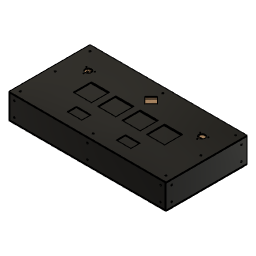
OpenSDVX Con v2 (Autodesk Fusion 360 design; units mm, degrees)
Autodesk Fusion 360 part; units mm, degrees
(part 1 of 2)
sketch "Bottom Panel Profile Sketch" plane through (0, 0, 0) normal (0, 1, 0) x (1, 0, 0) in component "Box"
  line L0 (245, 125) -> (-245, 125)
  line L1 (-245, 125) -> (-245, -125)
  line L2 (-245, -125) -> (245, -125)
  line L3 (245, -125) -> (245, 125)
  line L4 (245, 125) -> (-245, -125) construction
  line L5 (-245, 125) -> (245, -125) construction
  dimension "d31" = 490
  dimension "d32" = 250
  constraint horizontal L0
  constraint perpendicular L0 L1
  constraint parallel L0 L2
  constraint parallel L1 L3
  constraint coincident L4 origin
  constraint coincident L5 origin
  measures "d31" distance of L1.end L2.end
  measures "d32" distance of L0.end L1.end
extrude "Extrude1" add sketch "Bottom Panel Profile Sketch" along normal blind 6 makes body 1 in component "Box"
sketch "Bottom Panel Front Fingers Sketch" plane through (0, 0, 125) normal (0, 0, 1) x (1, 0, 0) in component "Box"
  line L0 (-245, 0) -> (245, 0)
  line L1 (245, 0) -> (245, 6)
  line L2 (245, 6) -> (-245, 6)
  line L3 (-245, 6) -> (-245, 0)
  line L4 (0, 6) -> (0, 0) construction
  line L5 (-232.4359, 3) -> (232.4359, 3) construction
  line L6 (-232.4359, 0) -> (-219.8718, 0)
  line L7 (-219.8718, 0) -> (-219.8718, 6)
  line L8 (-219.8718, 6) -> (-232.4359, 6)
  line L9 (-232.4359, 6) -> (-232.4359, 0)
  dimension "d35" = 12.5641
  dimension "d36" = 464.8718
  constraint midpoint L2 L4.start
  constraint coincident L4.end origin
  constraint perpendicular L4 L5
  constraint midpoint L4 L5
  constraint horizontal L6
  constraint vertical L7
  constraint horizontal L8
  constraint vertical L9
  constraint coincident L2 L7.end
  constraint coincident L0 L6.start
  constraint coincident L5.start L9
  measures "d35" distance of L7.end L8.end
  measures "d36" distance of L5.start L5.end
extrude "Extrude2" cut sketch "Bottom Panel Front Fingers Sketch" against normal blind 6 contours L0 L2 L6 L7 L8 L9 bodies 1 in component "Box"
pattern_linear "R-Pattern1" count 19 spacing 25.1282 along (1, 0, 0) count 2 spacing 244 along (0, 0, -1) of "Extrude2" in component "Box"
sketch "Bottom Panel Left Fingers Sketch" plane through (-245, 0, 0) normal (-1, 0, 0) x (0, 0, 1) in component "Box"
  line L0 (-125, 0) -> (125, 0)
  line L1 (125, 0) -> (125, 6)
  line L2 (125, 6) -> (-125, 6)
  line L3 (-125, 6) -> (-125, 0)
  line L4 (0, 6) -> (0, 0) construction
  line L5 (-111.8421, 3) -> (111.8421, 3) construction
  line L6 (98.6842, 0) -> (111.8421, 0)
  line L7 (111.8421, 0) -> (111.8421, 6)
  line L8 (111.8421, 6) -> (98.6842, 6)
  line L9 (98.6842, 6) -> (98.6842, 0)
  dimension "d43" = 13.1579
  dimension "d44" = 223.6842
  constraint midpoint L2 L4.start
  constraint coincident L4.end origin
  constraint perpendicular L4 L5
  constraint midpoint L4 L5
  constraint horizontal L6
  constraint vertical L7
  constraint horizontal L8
  constraint vertical L9
  constraint coincident L2 L7.end
  constraint coincident L0 L6.start
  constraint coincident L5.end L7
  measures "d43" distance of L6.start L6.end
  measures "d44" distance of L5.start L5.end
extrude "Extrude3" cut sketch "Bottom Panel Left Fingers Sketch" against normal blind 6 contours L0 L2 L6 L7 L8 L9 bodies 1 in component "Box"
pattern_linear "R-Pattern2" count 9 spacing 26.3158 along (0, 0, -1) count 2 spacing 484 along (1, 0, 0) of "Extrude3" in component "Box"
sketch "Front Panel Front Fingers Sketch" plane through (0, 0, 125) normal (0, 0, 1) x (1, 0, 0) in component "Box"
  line L0 (-232.4359, 0) -> (-232.4359, 6)
  line L1 (-232.4359, 6) -> (-245, 6)
  line L2 (-245, 6) -> (-245, 0)
  line L3 (-245, 0) -> (-232.4359, 0)
  line L4 (-245, 0) -> (245, 0)
  line L5 (245, 0) -> (245, 74)
  line L6 (245, 74) -> (-245, 74)
  line L7 (-245, 74) -> (-245, 0)
  dimension "d51" = 490
  dimension "d52" = 74
  constraint horizontal L4
  constraint vertical L5
  constraint horizontal L6
  constraint vertical L7
  constraint coincident L2.end L3.start
  measures "d51" distance of L2.end L4.end
  measures "d52" distance of L2.end L6.end
extrude "Extrude4" add sketch "Front Panel Front Fingers Sketch" against normal blind 6 separate body contours L0 L1 L4 L5 L6 L7 makes body 2 in component "Box"
combine "Combine1" operation cut target body 2 tool bodies 1 keep tools in component "Box"
sketch "Front Panel Left Finger Sketch" plane through (0, 0, 125) normal (0, 0, 1) x (1, 0, 0) in component "Box"
  line L0 (232.4359, 6) -> (245, 6)
  line L1 (245, 6) -> (245, 74)
  line L2 (245, 74) -> (-245, 74)
  line L3 (-245, 74) -> (-245, 6)
  line L4 (-245, 6) -> (-232.4359, 6)
  line L5 (-232.4359, 6) -> (-232.4359, 0)
  line L6 (-232.4359, 0) -> (-219.8718, 0)
  line L7 (-219.8718, 0) -> (-219.8718, 6)
  line L8 (-219.8718, 6) -> (-207.3077, 6)
  line L9 (-207.3077, 6) -> (-207.3077, 0)
  line L10 (-207.3077, 0) -> (-194.7436, 0)
  line L11 (-194.7436, 0) -> (-194.7436, 6)
  line L12 (-194.7436, 6) -> (-182.1795, 6)
  line L13 (-182.1795, 6) -> (-182.1795, 0)
  line L14 (-182.1795, 0) -> (-169.6154, 0)
  line L15 (-169.6154, 0) -> (-169.6154, 6)
  line L16 (-169.6154, 6) -> (-157.0513, 6)
  line L17 (-157.0513, 6) -> (-157.0513, 0)
  line L18 (-157.0513, 0) -> (-144.4872, 0)
  line L19 (-144.4872, 0) -> (-144.4872, 6)
  line L20 (-144.4872, 6) -> (-131.9231, 6)
  line L21 (-131.9231, 6) -> (-131.9231, 0)
  line L22 (-131.9231, 0) -> (-119.359, 0)
  line L23 (-119.359, 0) -> (-119.359, 6)
  line L24 (-119.359, 6) -> (-106.7949, 6)
  line L25 (-106.7949, 6) -> (-106.7949, 0)
  line L26 (-106.7949, 0) -> (-94.2308, 0)
  line L27 (-94.2308, 0) -> (-94.2308, 6)
  line L28 (-94.2308, 6) -> (-81.6667, 6)
  line L29 (-81.6667, 6) -> (-81.6667, 0)
  line L30 (-81.6667, 0) -> (-69.1026, 0)
  line L31 (-69.1026, 0) -> (-69.1026, 6)
  line L32 (-69.1026, 6) -> (-56.5385, 6)
  line L33 (-56.5385, 6) -> (-56.5385, 0)
  line L34 (-56.5385, 0) -> (-43.9744, 0)
  line L35 (-43.9744, 0) -> (-43.9744, 6)
  line L36 (-43.9744, 6) -> (-31.4103, 6)
  line L37 (-31.4103, 6) -> (-31.4103, 0)
  line L38 (-31.4103, 0) -> (-18.8462, 0)
  line L39 (-18.8462, 0) -> (-18.8462, 6)
  line L40 (-18.8462, 6) -> (-6.2821, 6)
  line L41 (-6.2821, 6) -> (-6.2821, 0)
  line L42 (-6.2821, 0) -> (6.2821, 0)
  line L43 (6.2821, 0) -> (6.2821, 6)
  line L44 (6.2821, 6) -> (18.8462, 6)
  line L45 (18.8462, 6) -> (18.8462, 0)
  line L46 (18.8462, 0) -> (31.4103, 0)
  line L47 (31.4103, 0) -> (31.4103, 6)
  line L48 (-245, 40) -> (-239, 40) construction
  line L49 (-242, 62.2) -> (-242, 17.8) construction
  line L50 (-245, 32.6) -> (-239, 32.6)
  line L51 (-239, 32.6) -> (-239, 17.8)
  line L52 (-239, 17.8) -> (-245, 17.8)
  line L53 (-245, 17.8) -> (-245, 32.6)
  line L54 (31.4103, 6) -> (43.9744, 6)
  line L55 (43.9744, 6) -> (43.9744, 0)
  line L56 (43.9744, 0) -> (56.5385, 0)
  line L57 (56.5385, 0) -> (56.5385, 6)
  line L58 (56.5385, 6) -> (69.1026, 6)
  line L59 (69.1026, 6) -> (69.1026, 0)
  line L60 (69.1026, 0) -> (81.6667, 0)
  line L61 (81.6667, 0) -> (81.6667, 6)
  line L62 (81.6667, 6) -> (94.2308, 6)
  line L63 (94.2308, 6) -> (94.2308, 0)
  line L64 (94.2308, 0) -> (106.7949, 0)
  line L65 (106.7949, 0) -> (106.7949, 6)
  line L66 (106.7949, 6) -> (119.359, 6)
  line L67 (119.359, 6) -> (119.359, 0)
  line L68 (119.359, 0) -> (131.9231, 0)
  line L69 (131.9231, 0) -> (131.9231, 6)
  line L70 (131.9231, 6) -> (144.4872, 6)
  line L71 (144.4872, 6) -> (144.4872, 0)
  line L72 (144.4872, 0) -> (157.0513, 0)
  line L73 (157.0513, 0) -> (157.0513, 6)
  line L74 (157.0513, 6) -> (169.6154, 6)
  line L75 (169.6154, 6) -> (169.6154, 0)
  line L76 (169.6154, 0) -> (182.1795, 0)
  line L77 (182.1795, 0) -> (182.1795, 6)
  line L78 (182.1795, 6) -> (194.7436, 6)
  line L79 (194.7436, 6) -> (194.7436, 0)
  line L80 (194.7436, 0) -> (207.3077, 0)
  line L81 (207.3077, 0) -> (207.3077, 6)
  line L82 (207.3077, 6) -> (219.8718, 6)
  line L83 (219.8718, 6) -> (219.8718, 0)
  line L84 (219.8718, 0) -> (232.4359, 0)
  line L85 (232.4359, 0) -> (232.4359, 6)
  dimension "d55" = 6
  dimension "d56" = 14.8
  dimension "d57" = 44.4
  constraint midpoint L3 L48.start
  constraint perpendicular L3 L48
  constraint perpendicular L48 L49
  constraint midpoint L48 L49
  constraint horizontal L50
  constraint vertical L51
  constraint horizontal L52
  constraint vertical L53
  constraint coincident L3 L50.start
  constraint coincident L49.end L52
  constraint coincident L48.end L51
  measures "d55" distance of L48.start L48.end
  measures "d56" distance of L50.start L52.end
  measures "d57" distance of L49.start L49.end
extrude "Extrude5" cut sketch "Front Panel Left Finger Sketch" against normal blind 6 contours L3 L50 L51 L52 L53 bodies 2 in component "Box"
pattern_linear "R-Pattern3" count 2 spacing 29.6 along (0, 1, 0) count 2 spacing 484 along (1, 0, 0) of "Extrude5" in component "Box"
pattern_linear "R-Pattern6" count 2 spacing 68 along (0, 1, 0) of bodies 1 makes body 3 in component "Box"
combine "Combine3" operation cut target body 2 tool bodies 3 keep tools in component "Box"
pattern_linear "R-Pattern7" count 2 spacing 244 along (0, 0, -1) of bodies 2 makes body 4 in component "Box"
sketch "Left Panel Profile Sketch" plane through (-245, 0, 0) normal (-1, 0, 0) x (0, 0, 1) in component "Box"
  line L0 (111.8421, 6) -> (111.8421, 0)
  line L1 (111.8421, 0) -> (125, 0)
  line L2 (125, 0) -> (125, 6)
  line L3 (125, 6) -> (111.8421, 6)
  line L4 (125, 0) -> (-125, 0)
  line L5 (-125, 0) -> (-125, 74)
  line L6 (-125, 74) -> (125, 74)
  line L7 (125, 74) -> (125, 0)
  dimension "d88" = 250
  dimension "d89" = 74
  constraint horizontal L4
  constraint vertical L5
  constraint horizontal L6
  constraint vertical L7
  constraint coincident L1.end L2.start
  measures "d88" distance of L1.end L4.end
  measures "d89" distance of L1.end L6.end
extrude "Extrude8" add sketch "Left Panel Profile Sketch" against normal blind 6 separate body contours L0 L3 L4 L5 L6 L7 makes body 5 in component "Box"
combine "Combine4" operation cut target body 5 tool bodies 3 2 4 1 keep tools in component "Box"
pattern_linear "R-Pattern8" count 2 spacing 484 along (1, 0, 0) of bodies 5 makes body 6 in component "Box"
sketch "Bottom Plate Profile Sketch" plane through (0, 0, 0) normal (0, 1, 0) x (1, 0, 0) in component "Box"
  line L0 (248, 128) -> (-248, 128)
  line L1 (-248, 128) -> (-248, -128)
  line L2 (-248, -128) -> (248, -128)
  line L3 (248, -128) -> (248, 128)
  line L4 (248, 128) -> (-248, -128) construction
  line L5 (-248, 128) -> (248, -128) construction
  dimension "d100" = 496
  dimension "d101" = 256
  constraint horizontal L0
  constraint perpendicular L0 L1
  constraint parallel L0 L2
  constraint parallel L1 L3
  constraint coincident L4 origin
  constraint coincident L5 origin
  measures "d100" distance of L1.end L2.end
  measures "d101" distance of L0.end L1.end
extrude "Extrude10" add sketch "Bottom Plate Profile Sketch" against normal blind 3 separate body makes body 7 in component "Box"
pattern_linear "R-Pattern9" count 2 spacing 77 along (0, 1, 0) of bodies 7 makes body 8 in component "Box"
sketch "Left Plate Profile Sketch" plane through (-245, 0, 0) normal (-1, 0, 0) x (0, -1, 0) in component "Box"
  line L0 (0, 0) -> (-74, 0) construction
  line L1 (-37, -125) -> (-37, 125) construction
  line L2 (-74, 128) -> (0, 128)
  line L3 (0, 128) -> (0, -128)
  line L4 (0, -128) -> (-74, -128)
  line L5 (-74, -128) -> (-74, 128)
  line L6 (-74, 128) -> (0, -128) construction
  line L7 (0, 128) -> (-74, -128) construction
  point P0 (-37, 0)
  dimension "d115" = 74
  dimension "d116" = 250
  dimension "d117" = 74
  dimension "d118" = 256
  constraint coincident L0.start origin
  constraint horizontal L0
  constraint vertical L1
  constraint midpoint L0 L1
  constraint horizontal L2
  constraint perpendicular L2 L3
  constraint parallel L2 L4
  constraint parallel L3 L5
  constraint coincident L6 P0
  constraint coincident L7 P0
  constraint midpoint L0 P0
  measures "d115" distance of L0.start L0.end
  measures "d116" distance of L1.start L1.end
  measures "d117" distance of L3.end L4.end
  measures "d118" distance of L2.end L3.end
extrude "Extrude12" add sketch "Left Plate Profile Sketch" along normal blind 3 separate body makes body 9 in component "Box"
pattern_linear "R-Pattern10" count 2 spacing 493 along (1, 0, 0) of bodies 9 makes body 10 in component "Box"
sketch "Front Plate Profile Sketch" plane through (0, 0, 0) normal (0, 0, 1) x (1, 0, 0) in component "Box"
  line L0 (0, 0) -> (0, 74) construction
  line L1 (-245, 37) -> (245, 37)
  line L2 (245, 74) -> (-245, 74)
  line L3 (-245, 74) -> (-245, 0)
  line L4 (-245, 0) -> (245, 0)
  line L5 (245, 0) -> (245, 74)
  line L6 (245, 74) -> (-245, 0) construction
  line L7 (-245, 74) -> (245, 0) construction
  point P0 (0, 37)
  dimension "d125" = 74
  dimension "d126" = 490
  dimension "d127" = 490
  dimension "d128" = 74
  constraint coincident L0.start origin
  constraint vertical L0
  constraint perpendicular L0 L1
  constraint midpoint L0 L1
  constraint horizontal L2
  constraint perpendicular L2 L3
  constraint parallel L2 L4
  constraint parallel L3 L5
  constraint coincident L6 P0
  constraint coincident L7 P0
  constraint midpoint L1 P0
  measures "d125" distance of L0.start L0.end
  measures "d126" distance of L1.start L1.end
  measures "d127" distance of L3.end L4.end
  measures "d128" distance of L2.end L3.end
extrude "Extrude13" add sketch "Front Plate Profile Sketch" along normal blind 3 from surface at 125 separate body makes body 11 in component "Box"
pattern_linear "R-Pattern11" count 2 spacing 253 along (0, 0, -1) of bodies 11 makes body 12 in component "Box"
sketch "Top Plate Screws Sketch" plane through (0, 77, 0) normal (0, 1, 0) x (-1, 0, 0) in component "Box"
  line L0 (-248, 128) -> (-248, -128)
  line L1 (-248, -128) -> (248, -128)
  line L2 (248, -128) -> (248, 128)
  line L3 (248, 128) -> (-248, 128)
  circle A0 centre (230, -110) radius 2.5
  circle A1 centre (0, -110) radius 2.5
  circle A2 centre (230, 0) radius 2.5
  line L4 (226, -112.3094) -> (230, -114.6188)
  line L5 (230, -114.6188) -> (234, -112.3094)
  line L6 (234, -112.3094) -> (234, -107.6906)
  line L7 (234, -107.6906) -> (230, -105.3812)
  line L8 (230, -105.3812) -> (226, -107.6906)
  line L9 (226, -107.6906) -> (226, -112.3094)
  line L10 (4, -107.6906) -> (0, -105.3812)
  line L11 (0, -105.3812) -> (-4, -107.6906)
  line L12 (-4, -107.6906) -> (-4, -112.3094)
  line L13 (-4, -112.3094) -> (0, -114.6188)
  line L14 (4, -112.3094) -> (4, -107.6906)
  line L15 (0, -114.6188) -> (4, -112.3094)
  line L16 (-226, -107.6906) -> (-230, -105.3812)
  line L17 (-230, -105.3812) -> (-234, -107.6906)
  line L18 (-234, -107.6906) -> (-234, -112.3094)
  line L19 (-234, -112.3094) -> (-230, -114.6188)
  line L20 (-226, -112.3094) -> (-226, -107.6906)
  line L21 (-230, -114.6188) -> (-226, -112.3094)
  line L22 (234, 2.3094) -> (230, 4.6188)
  line L23 (230, 4.6188) -> (226, 2.3094)
  line L24 (226, 2.3094) -> (226, -2.3094)
  line L25 (226, -2.3094) -> (230, -4.6188)
  line L26 (234, -2.3094) -> (234, 2.3094)
  line L27 (230, -4.6188) -> (234, -2.3094)
  line L28 (-226, 2.3094) -> (-230, 4.6188)
  line L29 (-230, 4.6188) -> (-234, 2.3094)
  line L30 (-234, 2.3094) -> (-234, -2.3094)
  line L31 (-234, -2.3094) -> (-230, -4.6188)
  line L32 (-226, -2.3094) -> (-226, 2.3094)
  line L33 (-230, -4.6188) -> (-226, -2.3094)
  line L34 (234, 112.3094) -> (230, 114.6188)
  line L35 (230, 114.6188) -> (226, 112.3094)
  line L36 (226, 112.3094) -> (226, 107.6906)
  line L37 (226, 107.6906) -> (230, 105.3812)
  line L38 (234, 107.6906) -> (234, 112.3094)
  line L39 (230, 105.3812) -> (234, 107.6906)
  line L40 (4, 112.3094) -> (0, 114.6188)
  line L41 (0, 114.6188) -> (-4, 112.3094)
  line L42 (-4, 112.3094) -> (-4, 107.6906)
  line L43 (-4, 107.6906) -> (0, 105.3812)
  line L44 (4, 107.6906) -> (4, 112.3094)
  line L45 (0, 105.3812) -> (4, 107.6906)
  line L46 (-226, 112.3094) -> (-230, 114.6188)
  line L47 (-230, 114.6188) -> (-234, 112.3094)
  line L48 (-234, 112.3094) -> (-234, 107.6906)
  line L49 (-234, 107.6906) -> (-230, 105.3812)
  line L50 (-226, 107.6906) -> (-226, 112.3094)
  line L51 (-230, 105.3812) -> (-226, 107.6906)
  circle A3 centre (-230, -110) radius 2.5
  circle A4 centre (-230, 0) radius 2.5
  circle A5 centre (230, 110) radius 2.5
  circle A6 centre (0, 110) radius 2.5
  circle A7 centre (-230, 110) radius 2.5
  point P0 (230, -110)
  dimension "d136" = 5
  dimension "d137" = 18
  dimension "d138" = 18
  dimension "d141" = -460
  dimension "d142" = 220
  dimension "d201" = 4
  dimension "d202" = 90
  dimension "d205" = -460
  dimension "d206" = 220
  constraint coincident P0 A0.centre
  measures "d136" diameter of A0
  measures "d137" distance of L2 P0
  measures "d138" distance of L1 P0
  measures "d201" distance of P0 L9
  measures "d202" angle of L1 L6
extrude "Extrude14" cut sketch "Top Plate Screws Sketch" against normal blind 9 contours A0 | A1 | A2 bodies 3 8 in component "Box"
extrude "Extrude15" cut sketch "Top Plate Screws Sketch" along normal blind 9 from surface at -80 contours A0 | A1 | A2 bodies 1 7 in component "Box"
sketch "Sketch1" plane through (-248, 0, 0) normal (-1, 0, 0) x (0, 0, 1)
  line L0 (-128, 74) -> (-128, 0)
  line L1 (-128, 0) -> (128, 0)
  line L2 (128, 0) -> (128, 74)
  line L3 (128, 74) -> (-128, 74)
sketch "Sketch2" plane through (-248, 37, 0) normal (-1, 0, 0) x (0, 0, 1)
sketch "Sketch3" plane through (-248, 0, 0) normal (-1, 0, 0) x (0, 0, 1)
  circle A0 centre (-110, 60) radius 2.5
  line L0 (-128, 74) -> (128, 74)
  line L1 (-128, 0) -> (-128, 74)
  line L2 (0, 74) -> (0, 0) construction
  line L3 (-128, 37) -> (128, 37) construction
  circle A1 centre (110, 60) radius 2.5
  circle A2 centre (-110, 14) radius 2.5
  circle A3 centre (110, 14) radius 2.5
  line L4 (128, 74) -> (-128, 74)
  line L5 (-105.9944, 62.2997) -> (-109.9888, 64.6188)
  line L6 (-109.9888, 64.6188) -> (-113.9944, 62.3191)
  line L7 (-113.9944, 62.3191) -> (-114.0056, 57.7003)
  line L8 (-114.0056, 57.7003) -> (-110.0112, 55.3812)
  line L9 (-110.0112, 55.3812) -> (-106.0056, 57.6809)
  line L10 (-106.0056, 57.6809) -> (-105.9944, 62.2997)
  line L11 (106.0056, 62.3191) -> (105.9944, 57.7003)
  line L12 (105.9944, 57.7003) -> (109.9888, 55.3812)
  line L13 (109.9888, 55.3812) -> (113.9944, 57.6809)
  line L14 (113.9944, 57.6809) -> (114.0056, 62.2997)
  line L15 (114.0056, 62.2997) -> (110.0112, 64.6188)
  line L16 (110.0112, 64.6188) -> (106.0056, 62.3191)
  line L17 (-113.9944, 16.3191) -> (-114.0056, 11.7003)
  line L18 (-114.0056, 11.7003) -> (-110.0112, 9.3812)
  line L19 (-110.0112, 9.3812) -> (-106.0056, 11.6809)
  line L20 (-106.0056, 11.6809) -> (-105.9944, 16.2997)
  line L21 (-105.9944, 16.2997) -> (-109.9888, 18.6188)
  line L22 (-109.9888, 18.6188) -> (-113.9944, 16.3191)
  line L23 (106.0056, 16.3191) -> (105.9944, 11.7003)
  line L24 (105.9944, 11.7003) -> (109.9888, 9.3812)
  line L25 (109.9888, 9.3812) -> (113.9944, 11.6809)
  line L26 (113.9944, 11.6809) -> (114.0056, 16.2997)
  line L27 (114.0056, 16.2997) -> (110.0112, 18.6188)
  line L28 (110.0112, 18.6188) -> (106.0056, 16.3191)
  point P0 (110, 60)
  point P1 (-110, 60)
  dimension "d148" = 5
  dimension "d149" = 14
  dimension "d150" = 18
  dimension "d151" = 74
  dimension "d152" = 256
  dimension "d155" = 220
  dimension "d156" = -46
  dimension "d186" = 220
  dimension "d187" = 46
  dimension "d195" = 4
  dimension "d196" = 0.139
  dimension "d199" = 220
  dimension "d200" = -46
  constraint midpoint L0 L2.start
  constraint coincident L2.end origin
  constraint perpendicular L2 L3
  constraint midpoint L2 L3
  constraint coincident P0 A1.centre
  constraint coincident A0.centre P1
  measures "d148" diameter of A0
  measures "d149" distance of A0.centre L0
  measures "d150" distance of A0.centre L1
  measures "d151" distance of L2.start L2.end
  measures "d152" distance of L3.start L3.end
  measures "d186" distance of A0.centre P0
  measures "d187" distance of A3.centre P0
  measures "d195" distance of P1 L10
  measures "d196" angle of L1 L7
extrude "Extrude16" cut sketch "Sketch3" against normal up to surface (496 mm away) contours A0 | A1 | A2 | A3 bodies 5 6 9 10 in component "Box"
sketch "Sketch4" plane through (0, 0, 128) normal (0, 0, 1) x (1, 0, 0)
  line L0 (245, 0) -> (245, 74)
  line L1 (245, 74) -> (-245, 74)
  line L2 (-245, 74) -> (-245, 0)
  line L3 (-245, 0) -> (245, 0)
  circle A0 centre (-231, 60) radius 2.5
  circle A1 centre (0, 60) radius 2.5
  circle A2 centre (231, 60) radius 2.5
  circle A3 centre (-231, 14) radius 2.5
  circle A4 centre (0, 14) radius 2.5
  circle A5 centre (231, 14) radius 2.5
  line L4 (-227.0014, 62.3118) -> (-231.0027, 64.6188)
  line L5 (-231.0027, 64.6188) -> (-235.0014, 62.307)
  line L6 (-235.0014, 62.307) -> (-234.9986, 57.6882)
  line L7 (-234.9986, 57.6882) -> (-230.9973, 55.3812)
  line L8 (-230.9973, 55.3812) -> (-226.9986, 57.693)
  line L9 (-226.9986, 57.693) -> (-227.0014, 62.3118)
  line L10 (-0.0027, 64.6188) -> (-4.0014, 62.307)
  line L11 (-4.0014, 62.307) -> (-3.9986, 57.6882)
  line L12 (-3.9986, 57.6882) -> (0.0027, 55.3812)
  line L13 (0.0027, 55.3812) -> (4.0014, 57.693)
  line L14 (4.0014, 57.693) -> (3.9986, 62.3118)
  line L15 (3.9986, 62.3118) -> (-0.0027, 64.6188)
  line L16 (230.9973, 64.6188) -> (226.9986, 62.307)
  line L17 (226.9986, 62.307) -> (227.0014, 57.6882)
  line L18 (227.0014, 57.6882) -> (231.0027, 55.3812)
  line L19 (231.0027, 55.3812) -> (235.0014, 57.693)
  line L20 (235.0014, 57.693) -> (234.9986, 62.3118)
  line L21 (234.9986, 62.3118) -> (230.9973, 64.6188)
  line L22 (-231.0027, 18.6188) -> (-235.0014, 16.307)
  line L23 (-235.0014, 16.307) -> (-234.9986, 11.6882)
  line L24 (-234.9986, 11.6882) -> (-230.9973, 9.3812)
  line L25 (-230.9973, 9.3812) -> (-226.9986, 11.693)
  line L26 (-226.9986, 11.693) -> (-227.0014, 16.3118)
  line L27 (-227.0014, 16.3118) -> (-231.0027, 18.6188)
  line L28 (-0.0027, 18.6188) -> (-4.0014, 16.307)
  line L29 (-4.0014, 16.307) -> (-3.9986, 11.6882)
  line L30 (-3.9986, 11.6882) -> (0.0027, 9.3812)
  line L31 (0.0027, 9.3812) -> (4.0014, 11.693)
  line L32 (4.0014, 11.693) -> (3.9986, 16.3118)
  line L33 (3.9986, 16.3118) -> (-0.0027, 18.6188)
  line L34 (230.9973, 18.6188) -> (226.9986, 16.307)
  line L35 (226.9986, 16.307) -> (227.0014, 11.6882)
  line L36 (227.0014, 11.6882) -> (231.0027, 9.3812)
  line L37 (231.0027, 9.3812) -> (235.0014, 11.693)
  line L38 (235.0014, 11.693) -> (234.9986, 16.3118)
  line L39 (234.9986, 16.3118) -> (230.9973, 18.6188)
  point P0 (-231, 60)
  dimension "d159" = 5
  dimension "d160" = 14
  dimension "d161" = 14
  dimension "d164" = 462
  dimension "d165" = -46
  dimension "d172" = 4
  dimension "d173" = 8
  dimension "d174" = 4
  dimension "d175" = 4
  dimension "d176" = 0.034
  dimension "d179" = 462
  dimension "d180" = -46
  constraint coincident P0 A0.centre
  measures "d159" diameter of A0
  measures "d160" distance of L1 P0
  measures "d161" distance of L2 P0
  measures "d172" distance of P0 L9
  measures "d173" distance of L6 L9
  measures "d174" distance of P0 L9
  measures "d175" distance of P0 L6
  measures "d176" angle of L2 L6
extrude "Extrude17" cut sketch "Sketch4" against normal up to surface (256 mm away) contours A0 | A1 | A2 | A3 | A4 | A5 bodies 2 11 12 in component "Box"
sketch "Sketch5" plane through (0, 0, 0) normal (0, -1, 0) x (1, 0, 0)
  circle A0 centre (0, -110) radius 2.5
  circle A1 centre (-230, -110) radius 2.5
  circle A2 centre (-230, 0) radius 2.5
  line L0 (239, -98.6842) -> (245, -98.6842)
  line L1 (245, -98.6842) -> (245, -85.5263)
  line L2 (245, -85.5263) -> (239, -85.5263)
  line L3 (239, -85.5263) -> (239, -72.3684)
  line L4 (239, -72.3684) -> (245, -72.3684)
  line L5 (245, -72.3684) -> (245, -59.2105)
  line L6 (245, -59.2105) -> (239, -59.2105)
  line L7 (239, -59.2105) -> (239, -46.0526)
  line L8 (239, -46.0526) -> (245, -46.0526)
  line L9 (245, -46.0526) -> (245, -32.8947)
  line L10 (245, -32.8947) -> (239, -32.8947)
  line L11 (239, -32.8947) -> (239, -19.7368)
  line L12 (239, -19.7368) -> (245, -19.7368)
  line L13 (245, -19.7368) -> (245, -6.5789)
  line L14 (245, -6.5789) -> (239, -6.5789)
  line L15 (239, -6.5789) -> (239, 6.5789)
  line L16 (239, 6.5789) -> (245, 6.5789)
  line L17 (245, 6.5789) -> (245, 19.7368)
  line L18 (245, 19.7368) -> (239, 19.7368)
  line L19 (239, 19.7368) -> (239, 32.8947)
  line L20 (239, 32.8947) -> (245, 32.8947)
  line L21 (245, 32.8947) -> (245, 46.0526)
  line L22 (245, 46.0526) -> (239, 46.0526)
  line L23 (239, 46.0526) -> (239, 59.2105)
  line L24 (239, 59.2105) -> (245, 59.2105)
  line L25 (245, 59.2105) -> (245, 72.3684)
  line L26 (245, 72.3684) -> (239, 72.3684)
  line L27 (239, 72.3684) -> (239, 85.5263)
  line L28 (239, 85.5263) -> (245, 85.5263)
  line L29 (245, 85.5263) -> (245, 98.6842)
  line L30 (245, 98.6842) -> (239, 98.6842)
  line L31 (239, 98.6842) -> (239, 111.8421)
  line L32 (239, 111.8421) -> (245, 111.8421)
  line L33 (245, 111.8421) -> (245, 125)
  line L34 (245, 125) -> (232.4359, 125)
  line L35 (232.4359, 125) -> (232.4359, 119)
  line L36 (232.4359, 119) -> (219.8718, 119)
  line L37 (219.8718, 119) -> (219.8718, 125)
  line L38 (219.8718, 125) -> (207.3077, 125)
  line L39 (207.3077, 125) -> (207.3077, 119)
  line L40 (207.3077, 119) -> (194.7436, 119)
  line L41 (194.7436, 119) -> (194.7436, 125)
  line L42 (194.7436, 125) -> (182.1795, 125)
  line L43 (182.1795, 125) -> (182.1795, 119)
  line L44 (182.1795, 119) -> (169.6154, 119)
  line L45 (169.6154, 119) -> (169.6154, 125)
  line L46 (169.6154, 125) -> (157.0513, 125)
  line L47 (157.0513, 125) -> (157.0513, 119)
  line L48 (157.0513, 119) -> (144.4872, 119)
  line L49 (144.4872, 119) -> (144.4872, 125)
  line L50 (144.4872, 125) -> (131.9231, 125)
  line L51 (131.9231, 125) -> (131.9231, 119)
  line L52 (131.9231, 119) -> (119.359, 119)
  line L53 (119.359, 119) -> (119.359, 125)
  line L54 (119.359, 125) -> (106.7949, 125)
  line L55 (106.7949, 125) -> (106.7949, 119)
  line L56 (106.7949, 119) -> (94.2308, 119)
  line L57 (94.2308, 119) -> (94.2308, 125)
  line L58 (94.2308, 125) -> (81.6667, 125)
  line L59 (81.6667, 125) -> (81.6667, 119)
  line L60 (81.6667, 119) -> (69.1026, 119)
  line L61 (69.1026, 119) -> (69.1026, 125)
  line L62 (69.1026, 125) -> (56.5385, 125)
  line L63 (56.5385, 125) -> (56.5385, 119)
  line L64 (56.5385, 119) -> (43.9744, 119)
  line L65 (43.9744, 119) -> (43.9744, 125)
  line L66 (43.9744, 125) -> (31.4103, 125)
  line L67 (31.4103, 125) -> (31.4103, 119)
  line L68 (31.4103, 119) -> (18.8462, 119)
  line L69 (18.8462, 119) -> (18.8462, 125)
  line L70 (18.8462, 125) -> (6.2821, 125)
  line L71 (6.2821, 125) -> (6.2821, 119)
  line L72 (6.2821, 119) -> (-6.2821, 119)
  line L73 (-6.2821, 119) -> (-6.2821, 125)
  line L74 (-6.2821, 125) -> (-18.8462, 125)
  line L75 (-18.8462, 125) -> (-18.8462, 119)
  line L76 (-18.8462, 119) -> (-31.4103, 119)
  line L77 (-31.4103, 119) -> (-31.4103, 125)
  line L78 (-31.4103, 125) -> (-43.9744, 125)
  line L79 (-43.9744, 125) -> (-43.9744, 119)
  line L80 (-43.9744, 119) -> (-56.5385, 119)
  line L81 (-56.5385, 119) -> (-56.5385, 125)
  line L82 (-56.5385, 125) -> (-69.1026, 125)
  line L83 (-69.1026, 125) -> (-69.1026, 119)
  line L84 (-69.1026, 119) -> (-81.6667, 119)
  line L85 (-81.6667, 119) -> (-81.6667, 125)
  line L86 (-81.6667, 125) -> (-94.2308, 125)
  line L87 (-94.2308, 125) -> (-94.2308, 119)
  line L88 (-94.2308, 119) -> (-106.7949, 119)
  line L89 (-106.7949, 119) -> (-106.7949, 125)
  line L90 (-106.7949, 125) -> (-119.359, 125)
  line L91 (-119.359, 125) -> (-119.359, 119)
  line L92 (-119.359, 119) -> (-131.9231, 119)
  line L93 (-131.9231, 119) -> (-131.9231, 125)
  line L94 (-131.9231, 125) -> (-144.4872, 125)
  line L95 (-144.4872, 125) -> (-144.4872, 119)
  line L96 (-144.4872, 119) -> (-157.0513, 119)
  line L97 (-157.0513, 119) -> (-157.0513, 125)
  line L98 (-157.0513, 125) -> (-169.6154, 125)
  line L99 (-169.6154, 125) -> (-169.6154, 119)
  line L100 (-169.6154, 119) -> (-182.1795, 119)
  line L101 (-182.1795, 119) -> (-182.1795, 125)
  line L102 (-182.1795, 125) -> (-194.7436, 125)
  line L103 (-194.7436, 125) -> (-194.7436, 119)
  line L104 (-194.7436, 119) -> (-207.3077, 119)
  line L105 (-207.3077, 119) -> (-207.3077, 125)
  line L106 (-207.3077, 125) -> (-219.8718, 125)
  line L107 (-219.8718, 125) -> (-219.8718, 119)
  line L108 (-219.8718, 119) -> (-232.4359, 119)
  line L109 (-232.4359, 119) -> (-232.4359, 125)
  line L110 (-232.4359, 125) -> (-245, 125)
  line L111 (-245, 125) -> (-245, 111.8421)
  line L112 (-245, 111.8421) -> (-239, 111.8421)
  line L113 (-239, 111.8421) -> (-239, 98.6842)
  line L114 (-239, 98.6842) -> (-245, 98.6842)
  line L115 (-245, 98.6842) -> (-245, 85.5263)
  line L116 (-245, 85.5263) -> (-239, 85.5263)
  line L117 (-239, 85.5263) -> (-239, 72.3684)
  line L118 (-239, 72.3684) -> (-245, 72.3684)
  line L119 (-245, 72.3684) -> (-245, 59.2105)
  line L120 (-245, 59.2105) -> (-239, 59.2105)
  line L121 (-239, 59.2105) -> (-239, 46.0526)
  line L122 (-239, 46.0526) -> (-245, 46.0526)
  line L123 (-245, 46.0526) -> (-245, 32.8947)
  line L124 (-245, 32.8947) -> (-239, 32.8947)
  line L125 (-239, 32.8947) -> (-239, 19.7368)
  line L126 (-239, 19.7368) -> (-245, 19.7368)
  line L127 (-245, 19.7368) -> (-245, 6.5789)
  line L128 (-245, 6.5789) -> (-239, 6.5789)
  line L129 (-239, 6.5789) -> (-239, -6.5789)
  line L130 (-239, -6.5789) -> (-245, -6.5789)
  line L131 (-245, -6.5789) -> (-245, -19.7368)
  line L132 (-245, -19.7368) -> (-239, -19.7368)
  line L133 (-239, -19.7368) -> (-239, -32.8947)
  line L134 (-239, -32.8947) -> (-245, -32.8947)
  line L135 (-245, -32.8947) -> (-245, -46.0526)
  line L136 (-245, -46.0526) -> (-239, -46.0526)
  line L137 (-239, -46.0526) -> (-239, -59.2105)
  line L138 (-239, -59.2105) -> (-245, -59.2105)
  line L139 (-245, -59.2105) -> (-245, -72.3684)
  line L140 (-245, -72.3684) -> (-239, -72.3684)
  line L141 (-239, -72.3684) -> (-239, -85.5263)
  line L142 (-239, -85.5263) -> (-245, -85.5263)
  line L143 (-245, -85.5263) -> (-245, -98.6842)
  line L144 (-245, -98.6842) -> (-239, -98.6842)
  line L145 (-239, -98.6842) -> (-239, -111.8421)
  line L146 (-239, -111.8421) -> (-245, -111.8421)
  line L147 (-245, -111.8421) -> (-245, -125)
  line L148 (-245, -125) -> (-232.4359, -125)
  line L149 (-232.4359, -125) -> (-232.4359, -119)
  line L150 (-232.4359, -119) -> (-219.8718, -119)
  line L151 (-219.8718, -119) -> (-219.8718, -125)
  line L152 (-219.8718, -125) -> (-207.3077, -125)
  line L153 (-207.3077, -125) -> (-207.3077, -119)
  line L154 (-207.3077, -119) -> (-194.7436, -119)
  line L155 (-194.7436, -119) -> (-194.7436, -125)
  line L156 (-194.7436, -125) -> (-182.1795, -125)
  line L157 (-182.1795, -125) -> (-182.1795, -119)
  line L158 (-182.1795, -119) -> (-169.6154, -119)
  line L159 (-169.6154, -119) -> (-169.6154, -125)
  line L160 (-169.6154, -125) -> (-157.0513, -125)
  line L161 (-157.0513, -125) -> (-157.0513, -119)
  line L162 (-157.0513, -119) -> (-144.4872, -119)
  line L163 (-144.4872, -119) -> (-144.4872, -125)
  line L164 (-144.4872, -125) -> (-131.9231, -125)
  line L165 (-131.9231, -125) -> (-131.9231, -119)
  line L166 (-131.9231, -119) -> (-119.359, -119)
  line L167 (-119.359, -119) -> (-119.359, -125)
  line L168 (-119.359, -125) -> (-106.7949, -125)
  line L169 (-106.7949, -125) -> (-106.7949, -119)
  line L170 (-106.7949, -119) -> (-94.2308, -119)
  line L171 (-94.2308, -119) -> (-94.2308, -125)
  line L172 (-94.2308, -125) -> (-81.6667, -125)
  line L173 (-81.6667, -125) -> (-81.6667, -119)
  line L174 (-81.6667, -119) -> (-69.1026, -119)
  line L175 (-69.1026, -119) -> (-69.1026, -125)
  line L176 (-69.1026, -125) -> (-56.5385, -125)
  line L177 (-56.5385, -125) -> (-56.5385, -119)
  line L178 (-56.5385, -119) -> (-43.9744, -119)
  line L179 (-43.9744, -119) -> (-43.9744, -125)
  line L180 (-43.9744, -125) -> (-31.4103, -125)
  line L181 (-31.4103, -125) -> (-31.4103, -119)
  line L182 (-31.4103, -119) -> (-18.8462, -119)
  line L183 (-18.8462, -119) -> (-18.8462, -125)
  line L184 (-18.8462, -125) -> (-6.2821, -125)
  line L185 (-6.2821, -125) -> (-6.2821, -119)
  line L186 (-6.2821, -119) -> (6.2821, -119)
  line L187 (6.2821, -119) -> (6.2821, -125)
  line L188 (6.2821, -125) -> (18.8462, -125)
  line L189 (18.8462, -125) -> (18.8462, -119)
  line L190 (18.8462, -119) -> (31.4103, -119)
  line L191 (31.4103, -119) -> (31.4103, -125)
  line L192 (31.4103, -125) -> (43.9744, -125)
  line L193 (43.9744, -125) -> (43.9744, -119)
  line L194 (43.9744, -119) -> (56.5385, -119)
  line L195 (56.5385, -119) -> (56.5385, -125)
  line L196 (56.5385, -125) -> (69.1026, -125)
  line L197 (69.1026, -125) -> (69.1026, -119)
  line L198 (69.1026, -119) -> (81.6667, -119)
  line L199 (81.6667, -119) -> (81.6667, -125)
  line L200 (81.6667, -125) -> (94.2308, -125)
  line L201 (94.2308, -125) -> (94.2308, -119)
  line L202 (94.2308, -119) -> (106.7949, -119)
  line L203 (106.7949, -119) -> (106.7949, -125)
  line L204 (106.7949, -125) -> (119.359, -125)
  line L205 (119.359, -125) -> (119.359, -119)
  line L206 (119.359, -119) -> (131.9231, -119)
  line L207 (131.9231, -119) -> (131.9231, -125)
  line L208 (131.9231, -125) -> (144.4872, -125)
  line L209 (144.4872, -125) -> (144.4872, -119)
  line L210 (144.4872, -119) -> (157.0513, -119)
  line L211 (157.0513, -119) -> (157.0513, -125)
  line L212 (157.0513, -125) -> (169.6154, -125)
  line L213 (169.6154, -125) -> (169.6154, -119)
  line L214 (169.6154, -119) -> (182.1795, -119)
  line L215 (182.1795, -119) -> (182.1795, -125)
  line L216 (182.1795, -125) -> (194.7436, -125)
  line L217 (194.7436, -125) -> (194.7436, -119)
  line L218 (194.7436, -119) -> (207.3077, -119)
  line L219 (207.3077, -119) -> (207.3077, -125)
  line L220 (207.3077, -125) -> (219.8718, -125)
  line L221 (219.8718, -125) -> (219.8718, -119)
  line L222 (219.8718, -119) -> (232.4359, -119)
  line L223 (232.4359, -119) -> (232.4359, -125)
  line L224 (232.4359, -125) -> (245, -125)
  line L225 (245, -125) -> (245, -111.8421)
  line L226 (245, -111.8421) -> (239, -111.8421)
  line L227 (239, -111.8421) -> (239, -98.6842)
  line L228 (220.5, 100.5) -> (-220.5, 100.5)
  line L229 (-220.5, 100.5) -> (-220.5, -100.5)
  line L230 (-220.5, -100.5) -> (220.5, -100.5)
  line L231 (220.5, -100.5) -> (220.5, 100.5)
  line L232 (220.5, 100.5) -> (-220.5, -100.5) construction
  line L233 (-220.5, 100.5) -> (220.5, -100.5) construction
  dimension "d168" = 441
  dimension "d169" = 201
  constraint horizontal L228
  constraint perpendicular L228 L229
  constraint parallel L228 L230
  constraint parallel L229 L231
  constraint coincident L232 origin
  constraint coincident L233 origin
  measures "d168" distance of L229.end L230.end
  measures "d169" distance of L228.end L229.end
extrude "Extrude18" cut sketch "Sketch5" against normal blind 6 contours L228 L229 L230 L231 bodies 1 in component "Box"
extrude "Extrude19" cut sketch "Sketch4" against normal up to surface (253 mm away) contours A0 | A1 | A2 | A3 | A4 | A5 | L4 L5 L6 L7 L8 L9 | L10 L11 L12 L13 L14 L15 | L16 L17 L18 L19 L20 L21 | L22 L23 L24 L25 L26 L27 | L28 L29 L30 L31 L32 L33 | L34 L35 L36 L37 L38 L39 bodies 2 4 in component "Box"
extrude "Extrude20" cut sketch "Sketch3" against normal up to surface (490 mm away) from surface at -3 contours A0 | A1 | A2 | A3 | L5 L6 L7 L8 L9 L10 | L11 L12 L13 L14 L15 L16 | L17 L18 L19 L20 L21 L22 | L23 L24 L25 L26 L27 L28 bodies 5 6 in component "Box"
extrude "Extrude21" cut sketch "Top Plate Screws Sketch" against normal up to surface (77 mm away) contours A0 | A1 | A2 | L4 L5 L6 L7 L8 L9 | L10 L11 L12 L13 L14 L15 | L16 L17 L18 L19 L20 L21 | L22 L23 L24 L25 L26 L27 | L28 L29 L30 L31 L32 L33 | L34 L35 L36 L37 L38 L39 | L40 L41 L42 L43 L44 L45 | L46 L47 L48 L49 L50 L51 | A3 | A4 | A5 | A6 | A7 bodies 1 3 in component "Box"
extrude "Extrude22" cut sketch "Top Plate Screws Sketch" against normal up to surface (80 mm away) contours A0 | A1 | A2 | A3 | A4 | A5 | A6 | A7 bodies 7 8 in component "Box"